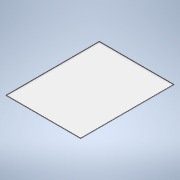
# Autodesk Inventor part: stol_1
Saved by Autodesk Inventor 2021 (Build 250183000, 183)
## iProperties
Created: 2022-03-11
Part Number: stol_1
Material: Generic
Document SubType Name: Modeling
Designer: Norbert_Prokopiuk
Mass: 6759 g
Surface Area: 65580 cm^2
Volume: 6759 cm^3
Density: 1 g/cm^3
Appearance: Default
Author: Norbert_Prokopiuk
Autodesk Inventor part; units mm, degrees
ref_plane "YZ Plane" through (0, 0, 0) normal (1, 0, 0) x (0, 1, 0)
ref_plane "XZ Plane" through (0, 0, 0) normal (0, 1, 0) x (-1, 0, 0)
ref_plane "XY Plane" through (0, 0, 0) normal (0, 0, 1) x (1, 0, 0)
sketch "Sketch1" plane through (0, 0, 0) normal (0, 1, 0) x (-1, 0, 0)
  line L0 (-800, 1000) -> (800, 1000)
  line L1 (800, 1000) -> (800, -1000)
  line L2 (800, -1000) -> (-800, -1000)
  line L3 (-800, -1000) -> (-800, 1000)
  line L4 (-800, 1000) -> (800, -1000) construction
  line L5 (800, 1000) -> (-800, -1000) construction
  point P0 (0, 0)
  dimension "d0" = 2000
  dimension "d1" = 1600
  constraints: 12 end point, 2 midpoint, 2 parallel, 1 horizontal, 1 perpendicular
  measures "d0" distance of L0.end L1.end
  measures "d1" distance of L0.start L0.end
extrude "Extrusion1" add sketch "Sketch1" along normal blind 12
sketch "Sketch2" plane through (0, 12, 0) normal (0, 1, 0) x (1, 0, 0)
  line L0 (-800, 1000) -> (-800, -1000) construction
  line L1 (-800, -1000) -> (800, -1000) construction
  line L2 (800, -1000) -> (800, 1000) construction
  line L3 (800, 1000) -> (-800, 1000) construction
  line L4 (-795, -995) -> (-795, 995)
  line L5 (-795, 995) -> (795, 995)
  line L6 (795, 995) -> (795, -995)
  line L7 (795, -995) -> (-795, -995)
  point P0 (0, 0)
  dimension "d4" = 5
  constraints: 8 end point, 3 other
  measures "d4" distance between parallel lines of L4 L0
extrude "Extrusion2" cut sketch "Sketch2" against normal blind 10
body "Solid1"
